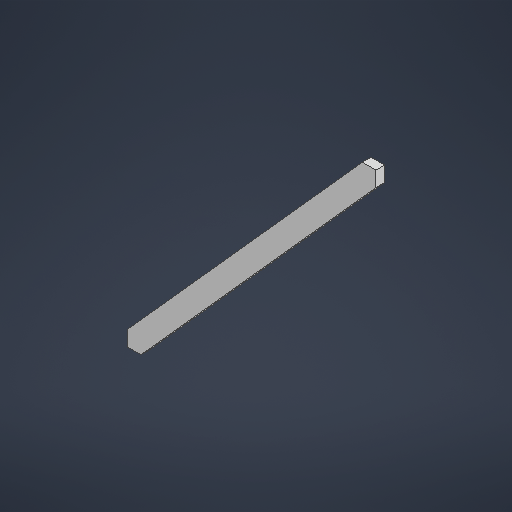
# Autodesk Inventor part: S_2x4x64.444
Saved by Autodesk Inventor 2026 (Build 300175000, 175)
## iProperties
Created: 2025-09-09
Part Number: S_2x4x64.444
Material: Generic
Document SubType Name: Modeling
Designer: trott
Density: 1 g/cm^3
Appearance: Default
Author: trott
Autodesk Inventor part; units mm, degrees
ref_plane "YZ Plane" through (0, 0, 0) normal (1, 0, 0) x (0, 1, 0)
ref_plane "XZ Plane" through (0, 0, 0) normal (0, 1, 0) x (-1, 0, 0)
ref_plane "XY Plane" through (0, 0, 0) normal (0, 0, 1) x (1, 0, 0)
sketch "Sketch1" plane through (0, 0, 0) normal (0, 0, 1) x (1, 0, 0)
  line L0 (-546.1, -609.6) -> (546.1, -609.6)
  line L1 (546.1, -609.6) -> (546.1, 609.6)
  line L2 (546.1, 609.6) -> (-546.1, 609.6)
  line L3 (-546.1, 609.6) -> (-546.1, -609.6)
  line L4 (-546.1, -609.6) -> (546.1, 609.6) construction
  line L5 (546.1, -609.6) -> (-546.1, 609.6) construction
  line L6 (546.1, 609.6) -> (-546.1, -609.6)
  line L7 (-512.9921, -639.2592) -> (-579.2079, -579.9408)
  line L8 (579.2079, 579.9408) -> (512.9921, 639.2592)
  line L9 (512.9921, 639.2592) -> (-579.2079, -579.9408)
  line L10 (579.2079, 579.9408) -> (-512.9921, -639.2592)
  point P0 (0, 0)
  point P1 (486.4224, 609.6)
  point P2 (-546.1, -542.9831)
  point P3 (-486.4224, -609.6)
  point P4 (546.1, 542.9831)
  dimension "d0" = 1092.2
  dimension "d1" = 1219.2
  dimension "d2" = 88.9
  dimension "d3" = 88.9
  constraints: 22 end point, 4 midpoint, 3 equal length, 3 perpendicular, 1 horizontal
  measures "d0" distance of L2.end L1.end
  measures "d1" distance of L0.end L1.end
  measures "d2" distance of L7.start L7.end
  measures "d3" distance of L8.start L8.end
extrude "Extrusion1" add sketch "Sketch1" along normal blind 38.1 contours L6 L1 L10 L0 | L3 L9 L2 L6
body "Solid1"
